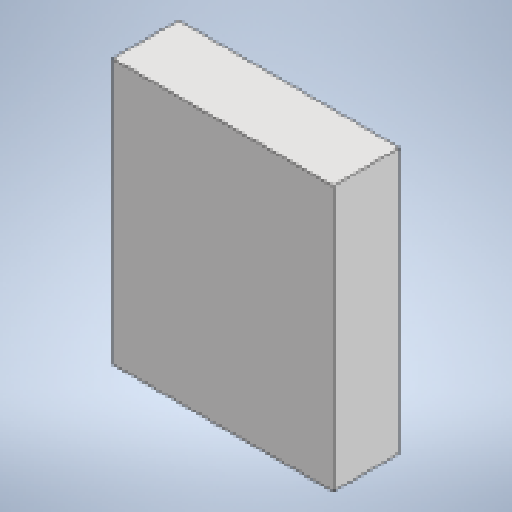
# Autodesk Inventor part: BSH 14 elactric
Saved by Autodesk Inventor 2025.1 (Build 291241020, 241B)
## iProperties
Created: 2024-08-27
Part Number: BSH 14 elactric
Material: Generic
Document SubType Name: Modeling
Designer: user
Density: 1 g/cm^3
Appearance: Default
Author: DELL
Autodesk Inventor part; units mm, degrees
ref_plane "YZ Plane" through (0, 0, 0) normal (1, 0, 0) x (0, 1, 0)
ref_plane "XZ Plane" through (0, 0, 0) normal (0, 1, 0) x (-1, 0, 0)
ref_plane "XY Plane" through (0, 0, 0) normal (0, 0, 1) x (1, 0, 0)
sketch "Sketch1" plane through (0, 0, 0) normal (0, 0, 1) x (1, 0, 0)
  line L0 (500, 150) -> (-500, 150)
  line L1 (-500, 150) -> (-500, -150)
  line L2 (-500, -150) -> (500, -150)
  line L3 (500, -150) -> (500, 150)
  line L4 (500, 150) -> (-500, -150) construction
  line L5 (-500, 150) -> (500, -150) construction
  point P0 (0, 0)
  dimension "d0" = 1000
  dimension "d1" = 300
  constraints: 12 end point, 2 midpoint, 2 parallel, 1 horizontal, 1 perpendicular
  measures "d0" distance of L2.end L1.end
  measures "d1" distance of L1.end L0.end
extrude "Extrusion1" add sketch "Sketch1" along normal blind 1200
body "Solid1"
